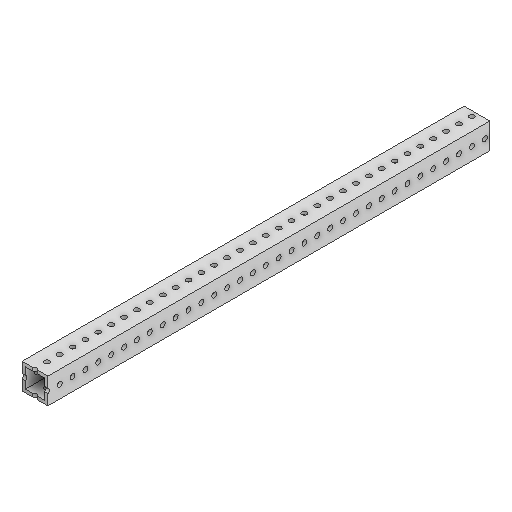
# Autodesk Inventor part: Move - Intake
Saved by Autodesk Inventor 2025.3 (Build 293356000, 356)
## iProperties
Created: 2026-05-13
Part Number: Move - Intake
Material: Genérico
Document SubType Name: Modeling
Designer: djair.oliveira
Density: 1 g/cm^3
Appearance: Padrão
Author: djair.oliveira
Autodesk Inventor part; units mm, degrees
ref_plane "YZ Plane" through (0, 0, 0) normal (1, 0, 0) x (0, 1, 0)
ref_plane "XZ Plane" through (0, 0, 0) normal (0, 1, 0) x (-1, 0, 0)
ref_plane "XY Plane" through (0, 0, 0) normal (0, 0, 1) x (1, 0, 0)
sketch "Esboço1" plane through (0, 0, 0) normal (1, 0, 0) x (0, 1, 0)
  line L0 (0, 0) -> (0, -435.695)
  line L1 (0, -435.695) -> (25.4, -435.695)
  line L2 (25.4, -435.695) -> (25.4, 0)
  line L3 (25.4, 0) -> (0, 0)
  line L4 (0, 0) -> (0, -435.695)
  circle A0 centre (12.7, -430.695) radius 2.5
  circle A1 centre (12.7, -417.995) radius 2.5
  circle A2 centre (12.7, -405.295) radius 2.5
  circle A3 centre (12.7, -392.595) radius 2.5
  circle A4 centre (12.7, -379.895) radius 2.5
  circle A5 centre (12.7, -367.195) radius 2.5
  circle A6 centre (12.7, -354.495) radius 2.5
  circle A7 centre (12.7, -341.795) radius 2.5
  circle A8 centre (12.7, -329.095) radius 2.5
  circle A9 centre (12.7, -316.395) radius 2.5
  circle A10 centre (12.7, -303.695) radius 2.5
  circle A11 centre (12.7, -290.995) radius 2.5
  circle A12 centre (12.7, -278.295) radius 2.5
  circle A13 centre (12.7, -265.595) radius 2.5
  circle A14 centre (12.7, -252.895) radius 2.5
  circle A15 centre (12.7, -240.195) radius 2.5
  circle A16 centre (12.7, -227.495) radius 2.5
  circle A17 centre (12.7, -214.795) radius 2.5
  circle A18 centre (12.7, -202.095) radius 2.5
  circle A19 centre (12.7, -189.395) radius 2.5
  circle A20 centre (12.7, -176.695) radius 2.5
  circle A21 centre (12.7, -163.995) radius 2.5
  circle A22 centre (12.7, -151.295) radius 2.5
  circle A23 centre (12.7, -138.595) radius 2.5
  circle A24 centre (12.7, -125.895) radius 2.5
  circle A25 centre (12.7, -113.195) radius 2.5
  circle A26 centre (12.7, -100.495) radius 2.5
  circle A27 centre (12.7, -87.795) radius 2.5
  circle A28 centre (12.7, -75.095) radius 2.5
  circle A29 centre (12.7, -62.395) radius 2.5
  circle A30 centre (12.7, -49.695) radius 2.5
  circle A31 centre (12.7, -36.995) radius 2.5
  circle A32 centre (12.7, -24.295) radius 2.5
  circle A33 centre (12.7, -11.595) radius 2.5
  circle A34 centre (12.7, 1.105) radius 2.5
  point P0 (14.9425, 0)
  point P1 (10.4575, 0)
  dimension "d1" = 435.695
  dimension "d2" = 25.4
  dimension "d3" = 5
  dimension "d4" = 12.7
  dimension "d5" = 5
  dimension "d8" = 12.7
  constraints: 35 centre point, 10 end point, 2 parallel, 2 vertical, 1 coincident, 1 horizontal, 1 perpendicular, 68 other
  measures "d1" distance of L0.start L0.end
  measures "d2" distance of L2.end L3.end
  measures "d3" diameter of A0
  measures "d4" distance from line of L2 A0.centre
  measures "d5" distance from line of L1 A0.centre
  measures "d8" distance of A0.centre A1.centre
extrude "Extrusão1" add sketch "Esboço1" along normal blind 25.4 contours L3 A34 L2 L1 L0
sketch "Esboço2" plane through (0, 0, -435.695) normal (0, 0, -1) x (-1, 0, 0)
  line L0 (-3.175, 3.175) -> (-22.225, 3.175)
  line L1 (-22.225, 3.175) -> (-22.225, 22.225)
  line L2 (-22.225, 22.225) -> (-3.175, 22.225)
  line L3 (-3.175, 22.225) -> (-3.175, 3.175)
  line L4 (0, 25.4) -> (-25.4, 25.4) projected
  line L5 (0, 0) -> (0, 25.4) projected
  line L6 (0, 0) -> (-25.4, 0) projected
  line L7 (-25.4, 0) -> (-25.4, 25.4) projected
  dimension "d15" = 3.175
  dimension "d16" = 3.175
  dimension "d17" = 3.175
  dimension "d18" = 3.175
  constraints: 8 end point, 2 parallel, 1 horizontal, 1 perpendicular
  measures "d15" distance between parallel lines of L4 L2
  measures "d16" distance between parallel lines of L5 L3
  measures "d17" distance between parallel lines of L6 L0
  measures "d18" distance between parallel lines of L7 L1
extrude "Extrusão2" cut sketch "Esboço2" against normal up to surface (435.695 mm away) contours L0 L1 L2 L3
sketch "Esboço3" plane through (0, 25.4, 0) normal (0, 1, 0) x (1, 0, 0)
  circle A0 centre (12.7, 430.695) radius 2.5
  line L0 (0, 435.695) -> (0, 0) projected
  line L1 (0, 435.695) -> (25.4, 435.695) projected
  circle A1 centre (12.7, 417.995) radius 2.5
  circle A2 centre (12.7, 405.295) radius 2.5
  circle A3 centre (12.7, 392.595) radius 2.5
  circle A4 centre (12.7, 379.895) radius 2.5
  circle A5 centre (12.7, 367.195) radius 2.5
  circle A6 centre (12.7, 354.495) radius 2.5
  circle A7 centre (12.7, 341.795) radius 2.5
  circle A8 centre (12.7, 329.095) radius 2.5
  circle A9 centre (12.7, 316.395) radius 2.5
  circle A10 centre (12.7, 303.695) radius 2.5
  circle A11 centre (12.7, 290.995) radius 2.5
  circle A12 centre (12.7, 278.295) radius 2.5
  circle A13 centre (12.7, 265.595) radius 2.5
  circle A14 centre (12.7, 252.895) radius 2.5
  circle A15 centre (12.7, 240.195) radius 2.5
  circle A16 centre (12.7, 227.495) radius 2.5
  circle A17 centre (12.7, 214.795) radius 2.5
  circle A18 centre (12.7, 202.095) radius 2.5
  circle A19 centre (12.7, 189.395) radius 2.5
  circle A20 centre (12.7, 176.695) radius 2.5
  circle A21 centre (12.7, 163.995) radius 2.5
  circle A22 centre (12.7, 151.295) radius 2.5
  circle A23 centre (12.7, 138.595) radius 2.5
  circle A24 centre (12.7, 125.895) radius 2.5
  circle A25 centre (12.7, 113.195) radius 2.5
  circle A26 centre (12.7, 100.495) radius 2.5
  circle A27 centre (12.7, 87.795) radius 2.5
  circle A28 centre (12.7, 75.095) radius 2.5
  circle A29 centre (12.7, 62.395) radius 2.5
  circle A30 centre (12.7, 49.695) radius 2.5
  circle A31 centre (12.7, 36.995) radius 2.5
  circle A32 centre (12.7, 24.295) radius 2.5
  circle A33 centre (12.7, 11.595) radius 2.5
  circle A34 centre (12.7, -1.105) radius 2.5
  dimension "d21" = 5
  dimension "d22" = 12.7
  dimension "d23" = 5
  dimension "d26" = 12.7
  constraints: 35 centre point, 1 vertical, 68 other
  measures "d21" diameter of A0
  measures "d22" distance from line of L0 A0.centre
  measures "d23" distance from line of L1 A0.centre
  measures "d26" distance of A0.centre A1.centre
extrude "Extrusão3" cut sketch "Esboço3" against normal up to surface (25.4 mm away)
equation "\"d16\" = d15"
equation "\"d17\" = d16"
equation "\"d18\" = d16"
